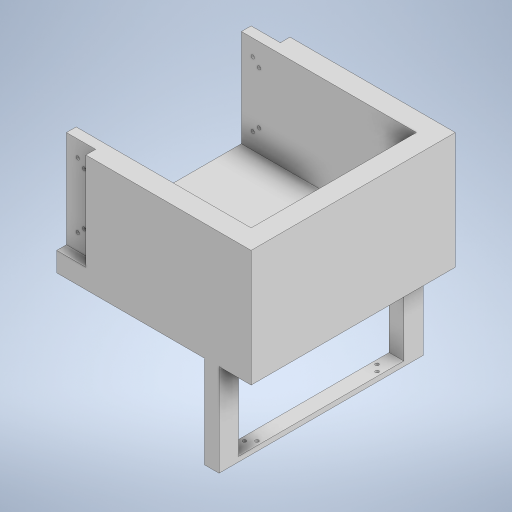
# Autodesk Inventor part: container_back
Saved by Autodesk Inventor 2023 (Build 270158000, 158)
## iProperties
Created: 2022-10-30
Part Number: container_back
Material: Genérico
Document SubType Name: Modeling
Designer: papel
Density: 1 g/cm^3
Appearance: Valor por defecto
Surface Area: 1564.19 cm^2
Author: papel
Autodesk Inventor part; units mm, degrees
ref_plane "YZ Plane" through (0, 0, 0) normal (1, 0, 0) x (0, 1, 0)
ref_plane "XZ Plane" through (0, 0, 0) normal (0, 1, 0) x (-1, 0, 0)
ref_plane "XY Plane" through (0, 0, 0) normal (0, 0, 1) x (1, 0, 0)
sketch "Boceto2" plane through (0, 0, 0) normal (0, 1, 0) x (-1, 0, 0)
  line L0 (7.5, 105) -> (-7.5, 105)
  line L1 (-7.5, 105) -> (-7.5, -105)
  line L2 (-7.5, -105) -> (7.5, -105)
  line L3 (7.5, -105) -> (7.5, 105)
  line L4 (7.5, 105) -> (-7.5, -105) construction
  line L5 (-7.5, 105) -> (7.5, -105) construction
  point P0 (0, 0)
  dimension "d7" = 15
  dimension "d8" = 210
  constraints: 12 end point, 2 midpoint, 2 parallel, 1 horizontal, 1 perpendicular
  measures "d7" distance of L2.end L1.end
  measures "d8" distance of L1.end L0.end
extrude "Extrusión1" add sketch "Boceto2" along normal blind 5
sketch "Boceto3" plane through (0, 5, 0) normal (0, 1, 0) x (1, 0, 0)
  line L0 (5, 60) -> (-5, 60)
  line L1 (-5, 60) -> (-5, 70)
  line L2 (-5, 70) -> (5, 70)
  line L3 (5, 70) -> (5, 60)
  line L4 (5, 60) -> (-5, 70) construction
  line L5 (7.5, 105) -> (-7.5, 105) projected
  line L6 (0, 64.5148) -> (0, 61.9205)
  circle A0 centre (3.25, 61.75) radius 1.75
  circle A1 centre (-3.25, 68.25) radius 1.75
  line L7 (-7.5, 105) -> (-7.5, -105) projected
  line L8 (-7.5, 0) -> (0, 0)
  line L9 (5, -70) -> (5, -60)
  line L10 (-5, -70) -> (5, -70)
  line L11 (5, -60) -> (-5, -60)
  line L12 (-5, -60) -> (-5, -70)
  line L13 (5, -60) -> (-5, -70) construction
  line L14 (0, -64.5148) -> (0, -61.9205)
  circle A2 centre (-3.25, -68.25) radius 1.75
  circle A3 centre (3.25, -61.75) radius 1.75
  point P0 (3.25, 68.25)
  point P1 (-5, 65)
  point P2 (-3.25, 61.75)
  point P3 (0, 105)
  point P4 (3.25, -68.25)
  point P5 (-3.25, -61.75)
  point P6 (-5, -65)
  dimension "d12" = 1.75
  dimension "d13" = 1.75
  dimension "d14" = 1.75
  dimension "d15" = 1.75
  dimension "d16" = 10
  dimension "d17" = 10
  dimension "d19" = 35
  dimension "d67" = 36.75
  constraints: 26 end point, 13 symmetric about line, 4 centre point, 3 midpoint, 2 horizontal, 2 parallel, 1 perpendicular, 1 vertical, 2 other
  measures "d12" distance from line of L2 point (3.25, 68.25)
  measures "d13" distance from line of L3 point (3.25, 68.25)
  measures "d14" distance from line of L1 point (-3.25, 61.75)
  measures "d15" distance from line of L0 point (-3.25, 61.75)
  measures "d16" distance between parallel lines of L0 L2
  measures "d17" distance between parallel lines of L3 L1
  measures "d19" distance from line of point (0, 105) L2
  measures "d67" distance from line of L5 A1.centre
hole "Agujero1" at (3.25, 5, -61.75) at (-3.25, 5, -68.25) at (-3.25, 5, 68.25) at (3.25, 5, 61.75) direction (0, -1, 0) diameter 3.5 end through all
sketch "Boceto4" plane through (0, 5, 0) normal (0, 1, 0) x (1, 0, 0)
  line L0 (-7.5, 105) -> (-7.5, -105) projected
  line L1 (-7.5, -105) -> (7.5, -105)
  line L2 (7.5, -105) -> (7.5, -85)
  line L3 (7.5, -85) -> (-7.5, -85)
  line L4 (-7.5, -85) -> (-7.5, -105)
  line L5 (-7.5, 0) -> (1.0116, 0)
  line L6 (-7.5, -105) -> (-7.5, 105)
  line L7 (-7.5, 105) -> (7.5, 105)
  line L8 (7.5, 105) -> (7.5, 85)
  line L9 (7.5, 85) -> (-7.5, 85)
  line L10 (-7.5, 85) -> (-7.5, 105)
  point P0 (0, 0)
  dimension "d27" = 15
  dimension "d28" = 20
  constraints: 20 end point, 5 symmetric about line, 2 horizontal, 2 parallel, 1 midpoint, 1 perpendicular
  measures "d27" distance of L3.end L2.end
  measures "d28" distance of L2.end L1.end
extrude "Extrusión2" add sketch "Boceto4" along normal blind 90
sketch "Boceto5" plane through (0, 95, 0) normal (0, 1, 0) x (1, 0, 0)
  line L0 (-7.5, -105) -> (7.5, -105) projected
  line L1 (-7.5, -105) -> (40.5, -105)
  line L2 (40.5, -105) -> (40.5, 105)
  line L3 (40.5, 105) -> (-7.5, 105)
  line L4 (-7.5, 105) -> (-7.5, -105)
  line L5 (40.5, -105) -> (-159.5, -105)
  line L6 (-159.5, -105) -> (-159.5, 105)
  line L7 (-159.5, 105) -> (40.5, 105)
  line L8 (40.5, 105) -> (40.5, -105)
  point P0 (0, 0)
  dimension "d31" = 48
  dimension "d32" = 200
  constraints: 16 end point, 4 parallel, 2 horizontal, 2 perpendicular, 1 point on line
  measures "d31" distance of L3.end L2.end
  measures "d32" distance of L6.end L7.end
extrude "Extrusión3" add sketch "Boceto5" along normal blind 120
sketch "Boceto6" plane through (0, 215, 0) normal (0, 1, 0) x (1, 0, 0)
  line L0 (40.5, 105) -> (7.5, 105) projected
  line L1 (40.5, 105) -> (20.5, 105)
  line L2 (20.5, 105) -> (20.5, 85)
  line L3 (7.5, -105) -> (40.5, -105) projected
  line L4 (24, -105) -> (24, -85)
  line L5 (-159.5, 105) -> (-159.5, -105) projected
  line L6 (20.5, 85) -> (-159.5, 85)
  line L7 (-159.5, 85) -> (-159.5, -85)
  line L8 (-159.5, -85) -> (20.5, -85)
  line L9 (20.5, -85) -> (20.5, 85)
  point P0 (7.5, 85)
  dimension "d36" = 20
  dimension "d37" = 20
  dimension "d38" = 20
  constraints: 14 end point, 2 parallel, 2 perpendicular, 2 point on line, 1 horizontal, 1 midpoint, 1 vertical
  measures "d36" distance of L0.start L1.end
  measures "d37" distance of L1.end L2.end
  measures "d38" distance of L4.start L4.end
extrude "Extrusión4" cut sketch "Boceto6" against normal blind 100
sketch "Boceto7" plane through (-159.5, 95, -105) normal (-1, 0, 0) x (0, 0, 1)
  line L0 (0, 120) -> (20, 120) projected
  line L1 (20, 120) -> (10, 120)
  line L2 (10, 120) -> (10, 20)
  line L3 (10, 20) -> (20, 20)
  line L4 (20, 20) -> (20, 120)
  line L5 (190, 120) -> (190, 20) projected
  line L6 (190, 120) -> (200, 120)
  line L7 (200, 120) -> (200, 20)
  line L8 (200, 20) -> (190, 20)
  line L9 (190, 20) -> (190, 120)
  line L10 (210, 0) -> (210, 120) projected
  line L11 (0, 0) -> (0, 120) projected
  line L12 (0, 120) -> (10, 120)
  line L13 (10, 120) -> (10, 20)
  line L14 (10, 20) -> (0, 20)
  line L15 (0, 20) -> (0, 120)
  line L16 (210, 120) -> (0, 120) projected
  line L17 (210, 120) -> (200, 120)
  line L18 (200, 120) -> (200, 20)
  line L19 (200, 20) -> (210, 20)
  line L20 (210, 20) -> (210, 120)
  point P0 (105, -95)
  dimension "d42" = 10
  dimension "d63" = 10
  dimension "d65" = 10
  constraints: 32 end point, 8 parallel, 4 horizontal, 4 perpendicular, 1 point on line
  measures "d42" distance of L7.end L8.end
  measures "d63" distance between parallel lines of L10 L7
  measures "d65" distance between parallel lines of L11 L2
extrude "Extrusión5" cut sketch "Boceto7" against normal blind 30 contours L0 L2 L14 L11 | L16 L10 L19 L7
sketch "Boceto8" plane through (-7.5, 0, 105) normal (0, 0, 1) x (1, 0, 0)
  line L0 (-122, 215) -> (-122, 115) projected
  line L1 (-132, 190) -> (-142, 190)
  line L2 (-142, 190) -> (-142, 200)
  line L3 (-142, 200) -> (-132, 200)
  line L4 (-132, 200) -> (-132, 190)
  line L5 (-132, 190) -> (-142, 200) construction
  line L6 (-142, 190) -> (-132, 200) construction
  line L7 (-152, 215) -> (48, 215) projected
  line L8 (-113, 165) -> (-128, 165)
  line L9 (-152, 115) -> (-122, 115) projected
  line L10 (-132, 195) -> (-131.5898, 195)
  circle A0 centre (-140.25, 198.25) radius 1.75
  circle A1 centre (-133.75, 191.75) radius 1.75
  line L11 (-132, 130) -> (-132, 140)
  line L12 (-142, 130) -> (-132, 130)
  line L13 (-132, 140) -> (-142, 130) construction
  line L14 (-132, 140) -> (-142, 140)
  line L15 (-142, 140) -> (-132, 130) construction
  line L16 (-142, 140) -> (-142, 130)
  line L17 (-132, 135) -> (-131.5898, 135)
  circle A2 centre (-133.75, 138.25) radius 1.75
  circle A3 centre (-140.25, 131.75) radius 1.75
  line L18 (-152, 115) -> (-152, 215) projected
  point P0 (7.5, 0)
  point P1 (-113, 215)
  point P2 (-133.75, 198.25)
  point P3 (-142, 195)
  point P4 (-140.25, 191.75)
  point P5 (-133.75, 131.75)
  point P6 (-140.25, 138.25)
  point P7 (-143, 115)
  point P8 (-133.75, 131.75)
  point P9 (-140.25, 138.25)
  point P10 (-142, 135)
  dimension "d46" = 1.75
  dimension "d47" = 1.75
  dimension "d48" = 1.75
  dimension "d49" = 1.75
  dimension "d50" = 10
  dimension "d51" = 10
  dimension "d52" = 15
  dimension "d66" = 10
  constraints: 30 end point, 15 symmetric about line, 4 centre point, 3 horizontal, 2 midpoint, 2 parallel, 1 perpendicular, 3 other
  measures "d46" distance from line of L3 point (-133.75, 198.25)
  measures "d47" distance from line of L4 point (-133.75, 198.25)
  measures "d48" distance from line of L2 point (-140.25, 191.75)
  measures "d49" distance from line of L1 point (-140.25, 191.75)
  measures "d50" distance between parallel lines of L1 L3
  measures "d51" distance between parallel lines of L4 L2
  measures "d52" distance between parallel lines of L7 L3
  measures "d66" distance between parallel lines of L18 L2
hole "Agujero2" at (-147.75, 198.25, 105) at (-141.25, 191.75, 105) at (-147.75, 131.75, 105) at (-141.25, 138.25, 105) direction (0, 0, -1) diameter 3.5 end through all
